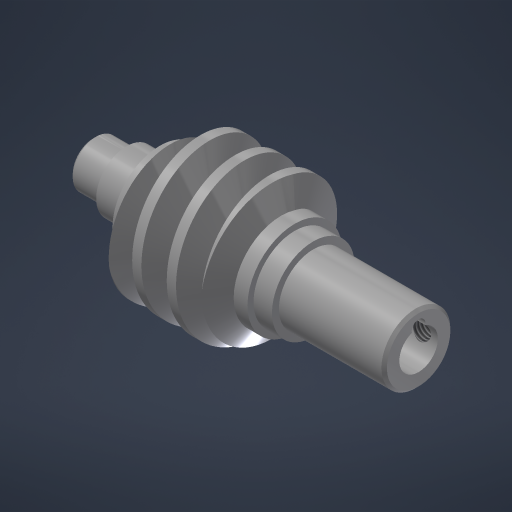
# Autodesk Inventor part: Worm
Saved by Autodesk Inventor 2023.1 (Build 271208000, 208)
## iProperties
CustomPartVersion: 1
Created: 2021-07-06
Part Number: Worm
Material: AISI 1045 - H
Document SubType Name: Modeling
Designer: Usuario
Categories: <?xml version="1.0" encoding="UTF-16"?> <MemberInstance><Categories><FamilyTemplate><FamilyTemplateParameter ValueType="xs:double" Id="1" ObjectReferenceKey="da_z" ObjectType="kUserParameterObject"/><FamilyTemplateParameter ValueType="xs:double" Id="2" ObjectReferenceKey="da_b" ObjectType="kUserParameterObject"/><FamilyTemplateParameter ValueType="xs:double" Id="3" ObjectReferenceKey="da_beta" ObjectType="kUserParameterObject"/><FamilyTemplateParameter ValueType="xs:double" Id="4" ObjectReferenceKey="da_m" ObjectType="kUserParameterObject"/><FamilyTemplateParameter ValueType="xs:double" Id="5" ObjectReferenceKey="da_alpha" ObjectType="kUserParameterObject"/><FamilyTemplateParameter ValueType="xs:double" Id="6" ObjectReferenceKey="da_da" ObjectType="kUserParameterObject"/><FamilyTemplateParameter ValueType="xs:double" Id="7" ObjectReferenceKey="da_aw" ObjectType="kUserParameterObject"/><FamilyTemplateParameter ValueType="xs:double" Id="8" ObjectReferenceKey="da_px" ObjectType="kUserParameterObject"/><FamilyTemplateParameter ValueType="xs:double" Id="9" ObjectReferenceKey="da_d" ObjectType="kUserParameterObject"/><FamilyTemplateParameter ValueType="xs:string" Id="10" ObjectReferenceKey="EAIAABAAAADKGAAAAAAAAIAAAAAAAAAA" ObjectType="83910656" SubObjectId="SurfaceGeometry"/></FamilyTemplate><ParamToTemplateMap><ParamToTemplate CategoryParameter="//CategoryParameter[@InternalName='046C89C9-8512-4d59-83FE-43B91F4F132A']" TemplateParameter="1"/><ParamToTemplate CategoryParameter="//CategoryParameter[@InternalName='2552DF32-E462-4b46-AEBF-C6C7768E72AC']" TemplateParameter="2"/><ParamToTemplate CategoryParameter="//CategoryParameter[@InternalName='C9EE641D-15FC-4fae-A226-E94C4372FDD7']" TemplateParameter="3"/><ParamToTemplate><ParamToTemplate CategoryParameter="//CategoryParameter[@InternalName='00B6519A-459B-49c7-AD84-2E56D39A5744']" ConstantValue="0.000000"/></ParamToTemplate><ParamToTemplate><ParamToTemplate CategoryParameter="//CategoryParameter[@InternalName='04B31F0E-C7A6-4894-AA32-9629BEFACF47']" ConstantValue="1.000000"/></ParamToTemplate><ParamToTemplate><ParamToTemplate CategoryParameter="//CategoryParameter[@InternalName='43CBEC2E-7847-49e7-A936-2F7889FCB2D9']" ConstantValue="0.200000"/></ParamToTemplate><ParamToTemplate><ParamToTemplate CategoryParameter="//CategoryParameter[@InternalName='B1EFC894-105D-4ebd-86BF-FA20ED196853']" ConstantValue="0.300000"/></ParamToTemplate><ParamToTemplate><ParamToTemplate CategoryParameter="//CategoryParameter[@InternalName='51175063-3D10-4879-93E8-6246FE8B403D']" ConstantValue="2067000000.000000"/></ParamToTemplate><ParamToTemplate><ParamToTemplate CategoryParameter="//CategoryParameter[@InternalName='A3A52E27-4454-46a9-B0BD-C932399B70AF']" ConstantValue="0.270000"/></ParamToTemplate><ParamToTemplate CategoryParameter="//CategoryParameter[@InternalName='91B76062-C214-41d9-B1B9-14D2AB99603D']" TemplateParameter="4"/><ParamToTemplate CategoryParameter="//CategoryParameter[@InternalName='2D373A89-B862-43d6-8D0B-0CBF12AB9F6C']" TemplateParameter="5"/><ParamToTemplate CategoryParameter="//CategoryParameter[@InternalName='37777632-D6A2-4fac-9D53-DB8ACD95C989']" TemplateParameter="6"/><ParamToTemplate CategoryParameter="//CategoryParameter[@InternalName='FD1017F1-B727-4f7e-9707-0F86F1FF9423']" TemplateParameter="7"/><ParamToTemplate CategoryParameter="//CategoryParameter[@InternalName='3BF567DA-17EF-48d8-80EA-D119B07F6463']" TemplateParameter="8"/><ParamToTemplate CategoryParameter="//CategoryParameter[@InternalName='BF5A1E7E-5373-4a22-AAD3-F583781FCF3C']" TemplateParameter="9"/><ParamToTemplate><ParamToTemplate CategoryParameter="//CategoryParameter[@InternalName='D4F72237-D604-435a-AD0B-F738B7463A00']" ConstantValue="1.000000"/></ParamToTemplate><ParamToTemplate CategoryParameter="//CategoryParameter[@InternalName='27C3BAF2-7550-4e4b-AE2C-0DB134B7D9B7']" TemplateParameter="10"/></ParamToTemplateMap><Category DisplayName="Gear" InternalName="DC85795E-93AB-48d5-8EEE-5A27447B64BD" Mnemonic="Gear"><CategoryParameter DisplayName="z" InternalName="046C89C9-8512-4d59-83FE-43B91F4F132A" Mnemonic="z"/><CategoryParameter DisplayName="b|.1|" InternalName="2552DF32-E462-4b46-AEBF-C6C7768E72AC" Mnemonic="b"/><CategoryParameter DisplayName="||g|" InternalName="C9EE641D-15FC-4fae-A226-E94C4372FDD7" Mnemonic="beta"/><CategoryParameter DisplayName="x" InternalName="00B6519A-459B-49c7-AD84-2E56D39A5744" Mnemonic="x"/><CategoryParameter DisplayName="a*" InternalName="04B31F0E-C7A6-4894-AA32-9629BEFACF47" Mnemonic="a"/><CategoryParameter DisplayName="c*" InternalName="43CBEC2E-7847-49e7-A936-2F7889FCB2D9" Mnemonic="c"/><CategoryParameter DisplayName="r|.f|*" InternalName="B1EFC894-105D-4ebd-86BF-FA20ED196853" Mnemonic="rf"/><CategoryParameter DisplayName="E" InternalName="51175063-3D10-4879-93E8-6246FE8B403D" Mnemonic="E"/><CategoryParameter DisplayName="||m|" InternalName="A3A52E27-4454-46a9-B0BD-C932399B70AF" Mnemonic="mi"/><Category DisplayName="WormGear" InternalName="1B25C7EF-093B-4025-B3D3-619CD2A4550C" Mnemonic="WormGear"><CategoryParameter DisplayName="m" InternalName="91B76062-C214-41d9-B1B9-14D2AB99603D" Mnemonic="m"/><CategoryParameter DisplayName="||a|" InternalName="2D373A89-B862-43d6-8D0B-0CBF12AB9F6C" Mnemonic="alpha"/><CategoryParameter DisplayName="d|.a|" InternalName="37777632-D6A2-4fac-9D53-DB8ACD95C989" Mnemonic="da"/><CategoryParameter DisplayName="a|.w|" InternalName="FD1017F1-B727-4f7e-9707-0F86F1FF9423" Mnemonic="aw"/><CategoryParameter DisplayName="p|.x|" InternalName="3BF567DA-17EF-48d8-80EA-D119B07F6463" Mnemonic="px"/><CategoryParameter DisplayName="d" InternalName="BF5A1E7E-5373-4a22-AAD3-F583781FCF3C" Mnemonic="d"/><CategoryParameter DisplayName="k|.mat|" InternalName="D4F72237-D604-435a-AD0B-F738B7463A00" Mnemonic="Coef"/><CategoryParameter DisplayName="PitchDiameter" InternalName="27C3BAF2-7550-4e4b-AE2C-0DB134B7D9B7" Mnemonic="IDS_PITCHDIAM"/></Category></Category></Categories></MemberInstance>
Density: 7.85 g/cm^3
Appearance: Steel(1)
Author: Usuario
Autodesk Inventor part; units mm, degrees
ref_plane "YZ Plane" through (0, 0, 0) normal (1, 0, 0) x (0, 1, 0)
ref_plane "XY Plane" through (0, 0, 0) normal (0, 0, 1) x (1, 0, 0)
sketch "Base Body Sketch" plane through (0, 0, 0) normal (1, 0, 0) x (0, 1, 0)
  circle A0 centre (0, 0) radius 26
  dimension "d5" = 52
extrude "Base Body" add sketch "Base Body Sketch" along normal mid plane 40
sketch "Sketch5" plane through (20, 0, 0) normal (1, 0, 0) x (0, 0, -1)
  circle A0 centre (0, 0) radius 26 projected
  circle A1 centre (0, 0) radius 22
  dimension "d59" = 44
  constraints: 1 centre point, 1 coincident
  measures "d59" diameter of A1
sketch "Sketch8" plane through (0, 0, 0) normal (0, 1, 0) x (-1, 0, 0)
  line L0 (-25, 17.2) -> (-25, -17.2) construction
  line L1 (24, -17.2) -> (24, 17.2) projected
  line L2 (272.4058, 0) -> (-272.4058, 0)
  line L3 (-25, 15) -> (-31.7, 15)
  line L4 (-31.7, 15) -> (-31.7, 12.5)
  line L5 (-31.7, 12.5) -> (-69.9, 12.5)
  line L6 (-69.9, 12.5) -> (-69.9, 0)
  line L7 (-69.9, 0) -> (-25, 0)
  line L8 (-25, 0) -> (-25, 15)
  point P0 (0, 0)
  point P1 (0, 0)
  dimension "d85" = 25
  dimension "d86" = 30
  dimension "d87" = 6.7
  dimension "d88" = 38.2
  constraints: 14 end point, 4 perpendicular, 3 point on line, 2 horizontal, 2 midpoint, 1 coincident
  measures "d85" diameter of L5 L2
  measures "d86" diameter of L3 L2
  measures "d87" distance of L3.start L3.end
  measures "d88" distance of L4.end L5.end
sketch "Sketch9" plane through (0, 0, 0) normal (0, 1, 0) x (-1, 0, 0)
  line L0 (24, -17.2) -> (24, 17.2) construction
  line L1 (105.0814, 0) -> (-105.0814, 0)
  line L2 (24, 11) -> (36.1, 11)
  line L3 (36.1, 11) -> (36.1, 8.5)
  line L4 (36.1, 8.5) -> (48.1, 8.5)
  line L5 (48.1, 8.5) -> (48.1, 0)
  line L6 (-69.9, -12.5) -> (-69.9, 12.5) projected
  line L7 (24, 11) -> (24, 0)
  line L8 (24, 0) -> (48.1, 0)
  point P0 (0, 0)
  point P1 (0, 0)
  dimension "d90" = 22
  dimension "d91" = 17
  dimension "d93" = 118
  dimension "d94" = 12
  constraints: 14 end point, 4 perpendicular, 3 point on line, 2 midpoint, 1 coincident, 1 collinear, 1 horizontal
  measures "d90" diameter of L2 L1
  measures "d91" diameter of L4 L1
  measures "d93" distance between parallel lines of L6 L5
  measures "d94" distance between parallel lines of L3 L5
surface extrude "Pitch Diameter" sketch "Sketch5" against normal through all shown no curves A1
chamfer "Chamfer1" distance 3.2029 distance2 8.8 1 edges at (20, -26, 0) measured on face at (19.5, -26, 0)
chamfer "Chamfer2" distance 3.2029 distance2 8.8 1 edges at (-20, -26, 0) measured on face at (-19.5, -26, 0)
sketch "Tooth Sketch" plane through (0, 0, 0) normal (0, 0, 1) x (1, 0, 0)
  line L0 (0, 21.74) -> (0, 10.96) projected
  line L1 (-36.108, 26.26) -> (-32.8105, 17.2)
  line L2 (-30.0214, 17.2) -> (-26.7238, 26.26)
  line L3 (-50.5346, 0) -> (-37.4554, 0) projected
  line L4 (-36.108, 26.26) -> (-31.4159, 26.26)
  line L5 (-31.4159, 26.26) -> (-26.7238, 26.26)
  line L6 (-32.8105, 17.2) -> (-31.4159, 17.2)
  line L7 (-31.4159, 17.2) -> (-30.0214, 17.2)
  line L8 (-31.4159, 22) -> (-28.2743, 22) construction
  line L9 (-31.4159, 26.26) -> (-31.4159, 17.2) construction
  dimension "d24" = 110
  dimension "d25" = 31.4159
  dimension "d26" = 3.1416
  dimension "d27" = 17.2
  dimension "d28" = 22
  dimension "d29" = 26.26
  constraints: 16 end point, 3 equal length, 3 parallel, 2 collinear, 2 point on line
  measures "d24" angle of L6 L1
  measures "d25" distance from line of L0 L4.end
  measures "d26" distance of L8.start L8.end
  measures "d27" distance between parallel lines of L3 L6
  measures "d28" distance between parallel lines of L3 L8
  measures "d29" distance between parallel lines of L3 L4
coil "Tooth" sketch "Tooth Sketch" operation cut axis through (-10, 0, 0) along (1, 0, 0) pitch 12.5664 turns 6 hand right
pattern_of_one "Tooth Pattern"
feature "Left Tooth" [suppressed]
pattern_circular "Left Tooth Pattern" [suppressed]
sketch "Sketch6" plane through (20, 0, 0) normal (1, 0, 0) x (0, 0, -1)
  arc A0 (2.094, 17.0721) -> (-16.4404, 5.0551) centre (0, 0) ccw projected
  arc A1 (-16.4404, 5.0551) -> (2.094, 17.0721) centre (0, 0) ccw projected
extrude "Extrusion2" add sketch "Sketch6" along normal blind 5
sketch "Sketch7" plane through (-20, 0, 0) normal (-1, 0, 0) x (0, 0, 1)
  arc A0 (2.094, 17.0721) -> (-16.4404, 5.0551) centre (0, 0) ccw projected
  arc A1 (-16.4404, 5.0551) -> (2.094, 17.0721) centre (0, 0) ccw projected
extrude "Extrusion3" add sketch "Sketch7" along normal blind 4 separate body
revolve "Revolution1" add sketch "Sketch8" angle 360 about axis through (-272.4058, 0, 0) along (1, 0, 0) separate body
revolve "Revolution2" add sketch "Sketch9" angle 360 about axis through (-105.0814, 0, 0) along (1, 0, 0) separate body
sketch "Sketch10" plane through (69.9, 0, 0) normal (1, 0, 0) x (0, 0, -1)
  point P0 (0, 0)
  point P1 (0, 0)
  constraints: 1 coincident
hole "Hole1" at (69.9, 0, 0) direction (-1, 0, 0) diameter 14 depth 40 tip angle 118 bodies 3
sketch "Sketch11" plane through (69.9, 0, 0) normal (1, 0, 0) x (0, 0, -1)
  circle A0 centre (0, 0) radius 7.1 construction
  circle A1 centre (-7.1, 0) radius 2.5
  circle A2 centre (0, 0) radius 7 construction
  point P0 (0, 7.1)
  point P1 (7, 0)
  point P2 (-9.6, 0)
  dimension "d104" = 5
  dimension "d121" = 16.6
  constraints: 5 horizontal alignment, 2 point on circle, 1 centre point, 1 coincident, 1 vertical alignment, 3 other
  measures "d121" distance of point (7, 0) point (-9.6, 0)
extrude "Extrusion4" cut sketch "Sketch11" against normal blind 32 bodies 3
ref_plane "Work Plane10" through (50.8, 12.5, 0) normal (0, 1, 0) x (-1, 0, 0)
sketch "Sketch12" plane through (50.8, 12.5, 0) normal (0, 1, 0) x (-1, 0, 0)
  line L0 (-19.1, -12.5) -> (-19.1, 12.5) projected
  point P0 (50.8, 0)
  point P1 (-13.35, 0)
  dimension "d107" = 5.75
  constraints: 1 horizontal alignment
  measures "d107" distance from line of L0 point (-13.35, 0)
hole "Hole2" at (64.15, 12.5, 0) direction (0, -1, 0) diameter 6.647 depth 12 tip angle 118 bodies 3 thread size "M8x1.25" class "6H" standard "ANSI Metric M Profile"
chamfer "Chamfer3" distance 1 angle 45 1 edges at (69.9, 0, -12.5)
chamfer "Chamfer4" distance 1 angle 45 1 edges at (-48.1, 0, -8.5)
scale "Scale1" factors (0.5, 0.5, 0.5) then translate (-15.025, 0, 0) bodies 4 2 1 3
equation "\"d6\" = da_b"
equation "\"d8\" = fd_cham1"
equation "\"d9\" = 0.5 * fd_cham2"
equation "\"d10\" = fd_cham1"
equation "\"d11\" = 0.5 * fd_cham2"
equation "\"d25\" = fd_dist"
equation "\"d26\" = 0.25 * da_px"
equation "\"d27\" = 0.5 * da_df"
equation "\"d28\" = 0.5 * da_d"
equation "\"d29\" = 0.505 * da_da"
equation "\"d32\" = fd_n"
equation "\"da_rightdir\" = 1"
equation "\"d64\" = fd_n"
equation "\"d5\" = da_da"
equation "\"d59\" = da_d"
equation "\"da_aw\" = 62"
equation "\"da_b\" = 40"
equation "\"da_df\" = 34.4"
equation "\"da_da\" = 52"
equation "\"fd_cham2\" = da_da - da_df"
equation "\"fd_cham1\" = 0.181985 * fd_cham2"
equation "\"da_d\" = 44"
equation "\"da_px\" = 12.566371"
equation "\"da_alfat\" = 20deg"
equation "\"d49\" = da_aw"
equation "\"d79\" = da_aw"
equation "\"fd_dist\" = 31.415927"
equation "\"fd_n\" = 6"
body "Solid1"
body "Srf1"
body "Solid2"
body "Solid3"
body "Solid4"
